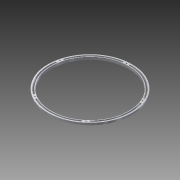
# Autodesk Inventor part: ytterring
Saved by Autodesk Inventor 2015 (Build 190159000, 159)
## iProperties
Created: 2015-02-04
Part Number: ytterring
Material: Generic
Document SubType Name: Modeling
Designer: janov_000
Density: 1 g/cm^3
Appearance: Aluminum - Flat
Author: janov_000
Autodesk Inventor part; units mm, degrees
ref_plane "YZ Plane" through (0, 0, 0) normal (1, 0, 0) x (0, 1, 0)
ref_plane "XZ Plane" through (0, 0, 0) normal (0, 1, 0) x (-1, 0, 0)
ref_plane "XY Plane" through (0, 0, 0) normal (0, 0, 1) x (1, 0, 0)
sketch "Sketch1" plane through (0, 0, 0) normal (0, 0, 1) x (1, 0, 0)
  circle A0 centre (0, 0) radius 162.5
  circle A1 centre (0, 0) radius 150
  line L0 (0, 0) -> (0, -162.5) construction
  dimension "outer_diameter" = 325
  dimension "inner_diameter" = 300
  constraints: 2 coincident, 2 end point, 1 centre point, 1 vertical, 1 vertical alignment, 2 other
  measures "inner_diameter" diameter of A1
extrude "Extrusion1" add sketch "Sketch1" along normal blind 10
sketch "Sketch2" plane through (0, 0, 10) normal (0, 0, 1) x (1, 0, 0)
  arc A0 (136.8569, 72.7681) -> (0, 155) centre (0, 0) ccw construction
  arc A1 (139.285, 74.0591) -> (0, 157.75) centre (0, 0) ccw
  arc A2 (134.4288, 71.477) -> (0, 152.25) centre (0, 0) ccw
  arc A3 (134.4288, 71.477) -> (139.285, 74.0591) centre (136.8569, 72.7681) ccw
  arc A4 (0, 157.75) -> (0, 152.25) centre (0, 155) ccw
  line L0 (0, 0) -> (136.8569, 72.7681) construction
  line L1 (0, 0) -> (0, 155) construction
  line L2 (0, 0) -> (0, -28.237) construction
  arc A5 (-27.393, 155.3534) -> (-150.0292, 48.7474) centre (0, 0) ccw
  arc A6 (-26.4379, 149.937) -> (-144.7984, 47.0478) centre (0, 0) ccw
  arc A7 (-26.4379, 149.937) -> (-27.393, 155.3534) centre (-26.9155, 152.6452) ccw
  arc A8 (-150.0292, 48.7474) -> (-144.7984, 47.0478) centre (-147.4138, 47.8976) ccw
  arc A9 (-156.2148, 21.9546) -> (-92.7231, -127.6224) centre (0, 0) ccw
  arc A10 (-150.7683, 21.1891) -> (-89.4903, -123.1728) centre (0, 0) ccw
  arc A11 (-150.7683, 21.1891) -> (-156.2148, 21.9546) centre (-153.4916, 21.5718) ccw
  arc A12 (-92.7231, -127.6224) -> (-89.4903, -123.1728) centre (-91.1067, -125.3976) ccw
  arc A13 (-69.153, -141.7848) -> (92.7231, -127.6224) centre (0, 0) ccw
  arc A14 (-66.742, -136.8414) -> (89.4903, -123.1728) centre (0, 0) ccw
  arc A15 (-66.742, -136.8414) -> (-69.153, -141.7848) centre (-67.9475, -139.3131) ccw
  arc A16 (92.7231, -127.6224) -> (89.4903, -123.1728) centre (91.1067, -125.3976) ccw
  arc A17 (113.4759, -109.5824) -> (150.0292, 48.7474) centre (0, 0) ccw
  arc A18 (109.5195, -105.7617) -> (144.7984, 47.0478) centre (0, 0) ccw
  arc A19 (109.5195, -105.7617) -> (113.4759, -109.5824) centre (111.4977, -107.672) ccw
  arc A20 (150.0292, 48.7474) -> (144.7984, 47.0478) centre (147.4138, 47.8976) ccw
  point P0 (162.5, 0)
  dimension "slot_radius" = 155
  dimension "slot_length_deg" = 62
  dimension "slot_width" = 5.5
  dimension "d15" = 360
  constraints: 42 point on circle, 21 centre point, 6 end point, 4 tangent, 1 coincident, 1 point on line, 1 vertical, 56 other
  measures "slot_radius" radius of A0
  measures "slot_length_deg" angle of L0 L1
  measures "slot_width" diameter of A3
extrude "Extrusion3" cut sketch "Sketch2" against normal blind 10
sketch "Sketch3" plane through (0, 0, 10) normal (0, 0, 1) x (1, 0, 0)
  circle A0 centre (0, 0) radius 150 projected
  circle A1 centre (0, 0) radius 155 construction
  line L0 (0, 0) -> (-13.5091, 154.4102) construction
  arc A2 (0, 157.75) -> (0, 152.25) centre (0, 155) ccw projected
  line L1 (0, 155) -> (0, 0) construction
  point P0 (-151.0274, 34.8674)
  point P1 (-79.8309, -132.8609)
  point P2 (101.6891, -116.98)
  point P3 (142.6783, 60.5633)
  dimension "d22" = 310
  dimension "d42" = 360
  dimension "d52" = 5
  constraints: 4 end point, 2 coincident, 9 other
  measures "d52" angle of L0 L1
hole "Hole1" at (-13.5091, 154.4102, 10) at (-151.0274, 34.8674, 10) at (-79.8309, -132.8609, 10) at (101.6891, -116.98, 10) at (142.6783, 60.5633, 10) direction (0, 0, -1) diameter 4.134 end through all thread size "M5x0.8" class "6H" standard "ANSI Metric M Profile"
sketch "Sketch5" plane through (0, 0, 0) normal (0, 0, -1) x (-1, 0, 0)
  circle A0 centre (0, 0) radius 162.5 projected
  circle A1 centre (0, 0) radius 160
  dimension "d53" = 320
  constraints: 1 centre point, 1 coincident
  measures "d53" diameter of A1
extrude "Extrusion4" cut sketch "Sketch5" against normal blind 8
equation "\"d17\" = thickness"
equation "\"offset_angle_gear\" = 65deg"
equation "\"thickness\" = 10"
body "Solid1"
